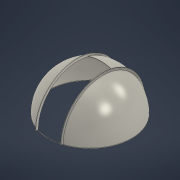
# Autodesk Inventor part: DomeHemisphere
Saved by Autodesk Inventor 2022 (Build 260153000, 153)
## iProperties
Created: 2021-05-07
Part Number: DomeHemisphere
Material: Generic
Document SubType Name: Modeling
Designer: Mick Veldhuis
Density: 1 g/cm^3
Appearance: Default
Author: Mick Veldhuis
Autodesk Inventor part; units mm, degrees
ref_plane "YZ Plane" through (0, 0, 0) normal (1, 0, 0) x (0, 1, 0)
ref_plane "XZ Plane" through (0, 0, 0) normal (0, 1, 0) x (-1, 0, 0)
sketch "Sketch6" plane through (0, 0, 0) normal (0, 1, 0) x (-1, 0, 0)
  circle A0 centre (0, 0) radius 3124
  circle A1 centre (0, 0) radius 3100
  constraints: 2 centre point, 2 coincident
extrude "Extrusion2" add sketch "Sketch6" along normal blind 40
ref_plane "Work Plane3" through (0, 40, 0) normal (0, 1, 0) x (1, 0, 0)
sketch "Sketch7" plane through (0, 40, 0) normal (0, 1, 0) x (1, 0, 0)
  line L0 (0, 3381) -> (0, -3319)
  line L1 (-3301, 0) -> (3261, 0)
  circle A0 centre (0, 0) radius 3100
  circle A1 centre (0, 0) radius 3124
  line L2 (920, -3124) -> (-920, -3124)
  line L3 (-920, -3124) -> (-920, 3124)
  line L4 (-920, 3124) -> (920, 3124)
  line L5 (920, 3124) -> (920, -3124)
  line L6 (920, -3124) -> (-920, 3124) construction
  line L7 (-920, -3124) -> (920, 3124) construction
  circle A2 centre (0, 0) radius 3100
  line L8 (-920, 2960.337819) -> (920, 2960.337819)
  line L9 (-920, -2960.337819) -> (920, -2960.337819)
  line L10 (960, -3124) -> (-960, -3124)
  line L11 (-960, -3124) -> (-960, 3124)
  line L12 (-960, 3124) -> (960, 3124)
  line L13 (960, 3124) -> (960, -3124)
  line L14 (960, -3124) -> (-960, 3124) construction
  line L15 (-960, -3124) -> (960, 3124) construction
  line L16 (960, -2947.609201) -> (-960, -2947.609201)
  point P0 (0, -3124)
  point P1 (0, -3100)
  point P2 (0, 3100)
  point P3 (0, 3124)
  point P4 (920, -2947.609201)
  point P5 (-920, -2947.609201)
  dimension "d12" = 1840
  constraints: 34 end point, 6 point on circle, 6 point on line, 4 midpoint, 4 parallel, 3 horizontal, 2 centre point, 2 coincident, 2 perpendicular, 1 vertical
  measures "d12" distance of L3.end L4.end
sketch "Sketch7 outline for Revolution4" plane through (0, 40, 0) normal (0, 1, 0) x (1, 0, 0)
  arc A0 (0, 3124) -> (0, -3124) centre (0, 0) ccw
  line L0 (0, 3100) -> (0, 3124)
  arc A1 (0, -3100) -> (0, 3100) centre (0, 0) cw
  line L1 (0, -3124) -> (0, -3100)
revolve "Revolution4" add sketch "Sketch7 outline for Revolution4" angle 180 about axis through (0, 40, -3381) along (0, 0, -1)
revolve "Revolution5" cut sketch "Sketch7" angle 105 about axis through (-3301, 40, 0) along (-1, 0, 0) picked at (895.128493, -2976.100487) picked at (-895.128493, -2976.100487) contours L9 A0 L0 | L0 A0 L9 | L5 A1 L0 A0 | A0 L0 A1 L3 | L5 L2 A1 | A1 L2 L3
revolve "Revolution6" add sketch "Sketch7" angle 180 about axis through (-3301, 40, 0) along (-1, 0, 0) picked at (928.901519, -2965.935467) picked at (-928.901519, -2965.935467) contours L16 A0 L5 | L3 A0 L16 | L13 L10 L5 A1 | A1 L5 A0 L13 | L11 A0 L3 A1 | A1 L3 L10 L11
body "Solid2"
